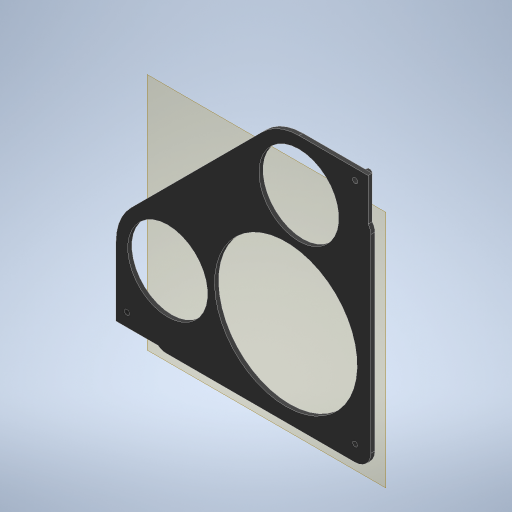
# Autodesk Inventor part: swerve protector
Saved by Autodesk Inventor 2023 (Build 270158030, 158C)
## iProperties
Created: 2022-07-21
Part Number: swerve protector
Material: Generic
Document SubType Name: Modeling
Designer: kt1040502
Density: 1 g/cm^3
Appearance: Default(1)
Author: kt1040502
Autodesk Inventor part; units mm, degrees
ref_plane "YZ Plane" through (0, 0, 0) normal (1, 0, 0) x (0, 1, 0)
ref_plane "XZ Plane" through (0, 0, 0) normal (0, 1, 0) x (-1, 0, 0)
ref_plane "XY Plane" through (0, 0, 0) normal (0, 0, 1) x (1, 0, 0)
ref_plane "Work Plane1" through (368.3, -368.3, 4.7625) normal (0, 0, 1) x (0, -1, 0)
sketch "Sketch1" plane through (368.3, -368.3, 4.7625) normal (0, 0, 1) x (0, -1, 0)
  spline S0 degree 3 number of poles 884
  arc A0 (-72.2824, -174.5174) -> (-43.815, -186.309) centre (-43.815, -146.05) ccw
  line L0 (-43.815, -186.309) -> (12.7, -186.309)
  line L1 (-174.5174, -72.2824) -> (-72.2824, -174.5174)
  arc A1 (-186.309, -43.815) -> (-174.5174, -72.2824) centre (-146.05, -43.815) ccw
  line L2 (-186.309, 12.7) -> (-186.309, -43.815)
  line L3 (-88.9, 10.16) -> (-647.7, 10.16)
  line L4 (10.16, -647.7) -> (10.16, -88.9)
  circle A2 centre (-43.815, -146.05) radius 31.1151
  circle A3 centre (-146.05, -43.815) radius 31.115
  line L5 (0, 0) -> (-123.3999, -123.3999) construction
  line L6 (0, -186.309) -> (0, 0) construction
  line L7 (0, 0) -> (-186.309, 0) construction
  spline S1 degree 3 number of poles 404 construction
  circle A4 centre (-53.9492, -53.9495) radius 55.5504
  line L8 (12.319, -147.6375) -> (12.319, -128.3493)
  line L9 (12.319, -125.6507) -> (12.319, -102.9776)
  line L10 (12.319, -748.919) -> (12.319, 12.7)
  line L11 (0, 12.319) -> (-53.975, 12.319)
  line L12 (-61.0927, 12.319) -> (-100.199, 12.319)
  line L13 (-147.6375, 12.319) -> (0, 12.319)
  arc A5 (12.319, 0) -> (0, 12.319) centre (0, 0) ccw
  arc A6 (-147.6375, 12.319) -> (-153.1614, 10.462) centre (-147.6375, 3.175) ccw
  arc A7 (-147.6375, 12.319) -> (-156.7815, 3.175) centre (-147.6375, 3.175) ccw
  line L14 (-156.7815, 3.175) -> (-156.7815, -3.175)
  arc A8 (-156.7815, -3.175) -> (-154.0017, -9.7408) centre (-147.6375, -3.175) ccw
  arc A9 (-156.7815, -3.175) -> (-147.6375, -12.319) centre (-147.6375, -3.175) ccw
  line L15 (-147.6375, -12.7) -> (-147.6375, -12.319)
  arc A10 (10.462, -153.1614) -> (12.319, -147.6375) centre (3.175, -147.6375) ccw
  arc A11 (3.175, -156.7815) -> (12.319, -147.6375) centre (3.175, -147.6375) ccw
  line L16 (-3.175, -156.7815) -> (3.175, -156.7815)
  arc A12 (-9.7408, -154.0017) -> (-3.175, -156.7815) centre (-3.175, -147.6375) ccw
  arc A13 (-12.319, -147.6375) -> (-3.175, -156.7815) centre (-3.175, -147.6375) ccw
  line L17 (-12.319, -147.6375) -> (-12.7, -147.6375)
  arc A14 (-175.7313, 0.0762) -> (-179.8687, 0.0762) centre (-177.8, 0) ccw
  arc A15 (-179.8687, -0.0762) -> (-175.7313, -0.0762) centre (-177.8, 0) ccw
  arc A16 (-0.0762, -175.7313) -> (-0.0762, -179.8687) centre (0, -177.8) ccw
  arc A17 (0.0762, -179.8687) -> (0.0762, -175.7313) centre (0, -177.8) ccw
  line L18 (-147.6375, 12.319) -> (-186.309, 12.319)
  line L19 (-147.6375, 12.319) -> (0, 12.319)
  line L20 (-186.309, 12.319) -> (-186.309, -43.815)
  line L21 (12.319, -186.309) -> (12.319, 0)
  line L22 (-174.5174, -72.2824) -> (-72.2824, -174.5174)
  line L23 (12.319, -186.309) -> (-43.815, -186.309)
  arc A18 (-72.2824, -174.5174) -> (-43.815, -186.309) centre (-43.815, -146.05) ccw
  arc A19 (-186.309, -43.815) -> (-174.5174, -72.2824) centre (-146.05, -43.815) ccw
  arc A20 (12.319, 0) -> (-0.0762, 12.319) centre (-0.0004, -0.0002) ccw
  circle A21 centre (-0.0004, -0.0002) radius 1.8977
  circle A22 centre (-177.8, 0) radius 2.0701
  circle A23 centre (0, -177.8) radius 2.0701
  point P0 (-368.3, -368.3)
  point P1 (-153.5386, 10.16)
  point P2 (-186.309, 10.16)
  point P3 (10.16, -186.309)
  point P4 (10.16, -153.5386)
  point P5 (7.669, 9.6408)
  point P6 (-179.8687, -0.0762)
  point P7 (-179.8687, 0.0762)
  point P8 (-175.7313, 0.0762)
  point P9 (-175.7313, -0.0762)
  point P10 (0.0762, -179.8687)
  point P11 (-0.0762, -179.8687)
  point P12 (-0.0762, -175.7313)
  point P13 (0.0762, -175.7313)
  constraints: 18 end point, 9 centre point, 7 tangent, 6 point on circle, 6 point on line, 5 coincident, 4 collinear, 2 concentric, 2 perpendicular, 1 midpoint, 1 parallel
extrude "Extrusion1" add sketch "Sketch1" along normal blind 3.175 contours L1 A1 L2 L3 A7 A6 L13 L12 L11 A5 L10 L9 L8 A10 A11 L4 L0 A0
sketch "Sketch2" plane through (368.3, -368.3, 4.7625) normal (0, 0, -1) x (-1, 0, 0)
  circle A0 centre (177.8, 0) radius 2.0701 projected
  circle A1 centre (177.8, 0) radius 2.0701
  circle A2 centre (0, 177.8) radius 2.0701 projected
  circle A3 centre (0, 177.8) radius 2.0701
  circle A4 centre (177.8, 0) radius 2.54
  circle A5 centre (0, 177.8) radius 2.54
  point P0 (368.3, 368.3)
  dimension "d2" = 5.08
  dimension "d3" = 5.08
  constraints: 4 centre point, 4 coincident
  measures "d2" diameter of A4
  measures "d3" diameter of A5
extrude "Extrusion2" add sketch "Sketch2" along normal blind 7.9502
body "Solid1"
